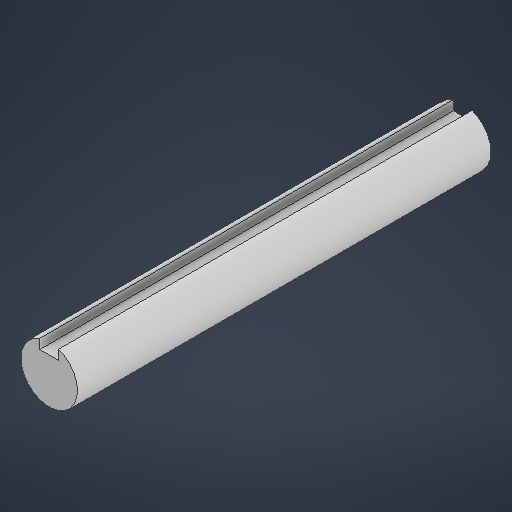
# Autodesk Inventor part: shaft_with_keyway
Saved by Autodesk Inventor 2026.1 (Build 301233000, 233)
## iProperties
Created: 2025-03-08
Part Number: shaft_with_keyway
Material: Generic
Document SubType Name: Modeling
Designer: aaron
Density: 1 g/cm^3
Appearance: Default
Author: aaron
Autodesk Inventor part; units mm, degrees
ref_plane "YZ Plane" through (0, 0, 0) normal (1, 0, 0) x (0, 1, 0)
ref_plane "XZ Plane" through (0, 0, 0) normal (0, 1, 0) x (-1, 0, 0)
ref_plane "XY Plane" through (0, 0, 0) normal (0, 0, 1) x (1, 0, 0)
sketch "Sketch1" plane through (0, 0, 0) normal (0, 0, 1) x (1, 0, 0)
  circle A0 centre (0, 0) radius 7.5
  line L0 (0, 7.5) -> (-2.5, 7.5)
  line L1 (-2.5, 7.5) -> (-2.5, 4.5)
  line L2 (-2.5, 4.5) -> (0, 4.5)
  line L3 (0, 4.5) -> (0, 7.5)
  line L4 (0, 7.5) -> (2.5, 7.5)
  line L5 (2.5, 7.5) -> (2.5, 4.5)
  line L6 (2.5, 4.5) -> (0, 4.5)
  point P0 (-2.5, 7.0711)
  point P1 (2.5, 7.0711)
  dimension "d0" = 15
  dimension "d1" = 3
  dimension "d2" = 2.5
  constraints: 14 end point, 2 parallel, 2 symmetric about line, 1 coincident, 1 horizontal, 1 perpendicular, 3 other
  measures "d1" distance of L0.end L1.end
  measures "d2" distance of L1.end L2.end
extrude "Extrusion1" add sketch "Sketch1" along normal blind 110 contours A0 L1 L2 L6 L5
body "Solid1"
